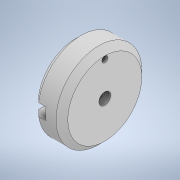
# Autodesk Inventor part: 711134
Saved by Autodesk Inventor 2022 (Build 260153000, 153)
## iProperties
Created: 2021-10-22
Part Number: 711134
Material: Типовые
Document SubType Name: Modeling
Designer: RaNSiD
Density: 1 g/cm^3
Appearance: По умолчанию
Mass: 20.8625 g
Surface Area: 65.1231 cm^2
Volume: 20.8625 cm^3
Author: RaNSiD
Autodesk Inventor part; units mm, degrees
ref_plane "YZ Plane" through (0, 0, 0) normal (1, 0, 0) x (0, 1, 0)
ref_plane "XZ Plane" through (0, 0, 0) normal (0, 1, 0) x (-1, 0, 0)
ref_plane "XY Plane" through (0, 0, 0) normal (0, 0, 1) x (1, 0, 0)
sketch "Эскиз5" plane through (0, 0, 0) normal (0, 0, 1) x (1, 0, 0)
  line L0 (0, 0) -> (20, 0)
  line L1 (20, 0) -> (20, 25)
  line L2 (16, 29) -> (4, 29)
  line L3 (0, 25) -> (0, 0)
  line L4 (4, 29) -> (0, 25)
  line L5 (16, 29) -> (20, 25)
  point P0 (20, 29)
  point P1 (0, 29)
  dimension "d33" = 20
  dimension "d34" = 29
  dimension "d35" = 4
  dimension "d36" = 4
  dimension "d37" = 4
  dimension "d38" = 4
  constraints: 12 end point, 4 point on line, 2 parallel, 1 horizontal, 1 perpendicular
  measures "d33" distance of point (0, 29) point (20, 29)
  measures "d34" distance of point (20, 29) L0.end
  measures "d35" distance of L2.end point (0, 29)
  measures "d36" distance of L3.start point (0, 29)
  measures "d37" distance of L2.start point (20, 29)
  measures "d38" distance of L1.end point (20, 29)
revolve "Вращение3" add sketch "Эскиз5" angle 360 about axis through (0, 0, 0) along (1, 0, 0)
sketch "Эскиз6" plane through (0, 0, 0) normal (0, 0, 1) x (1, 0, 0)
  line L0 (0, -25) -> (0, 25) construction
  line L1 (0, 4) -> (9, 4)
  line L2 (9, 4) -> (9, -4)
  line L3 (9, -4) -> (0, -4)
  line L4 (0, -4) -> (0, 4)
  point P0 (0, 0)
  point P1 (0, 0)
  point P2 (0, 0)
  dimension "d40" = 9
  dimension "d41" = 8
  constraints: 8 end point, 2 midpoint, 2 parallel, 1 coincident, 1 horizontal, 1 perpendicular, 1 point on line
  measures "d40" distance of L2.end L3.end
  measures "d41" distance of L1.end L2.end
extrude "Выдавливание2" cut sketch "Эскиз6" along normal through all both and the other way through all
sketch "Эскиз7" plane through (0, 0, 0) normal (-1, 0, 0) x (0, 0, 1)
  line L0 (0, 0) -> (0, 23) construction
  dimension "d44" = 23
  constraints: 2 end point, 1 coincident, 1 vertical
  measures "d44" distance of L0.start L0.end
hole "Отверстие2" at (0, 23, 0) direction (1, 0, 0) diameter 4 end through all
sketch "Эскиз8" plane through (20, 0, 0) normal (1, 0, 0) x (0, 0, -1)
  point P0 (0, 0)
  point P1 (0, 0)
  constraints: 1 coincident
hole "Отверстие3" at (20, 0, 0) direction (-1, 0, 0) diameter 8 depth 5
sketch "Эскиз9" plane through (15, 0, 0) normal (1, 0, 0) x (0, 0, -1)
  circle A0 centre (0, 0) radius 4.5
  dimension "d59" = 9
  constraints: 1 centre point, 1 coincident
  measures "d59" diameter of A0
extrude "Выдавливание3" cut sketch "Эскиз9" against normal blind 0.5
thread "Резьба2" size "M8x1.25" class "6H" standard "ANSI Metric M Profile" full length
equation "\"d36\" = d35"
equation "\"d37\" = d35"
equation "\"d38\" = d37"
